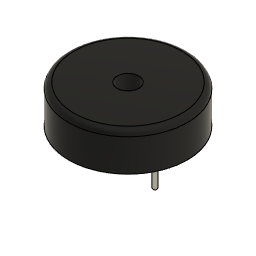
ManvirExam v2 (Autodesk Fusion 360 archive; units mm, degrees)
design "PKM22EPPH4001-B0"
Autodesk Fusion 360 part; units mm, degrees
ref_plane "WorkPlane1" through (0, 0, 1.2) normal (0, 0, 1) x (1, 0, 0) in component "Body"
sketch "Sketch1" plane through (0, 0, 1.2) normal (0, 0, 1) x (1, 0, 0) in component "Body"
  circle A0 centre (0, 0) radius 11
  dimension "d2" = 22
  constraint coincident A0.centre origin
  measures "d2" diameter of A0
extrude "Extrude1" add sketch "Sketch1" along normal blind 7 makes body 1 in component "Body"
fillet "Fillet1" radius 1 1 edges at (-10.2556, -3.9778, 8.2) on bodies 1 in component "Body"
sketch "Sketch2" plane through (0, 0, 1.2) normal (0, 0, -1) x (1, 0, 0) in component "Body"
  circle A0 centre (0, 0) radius 11
  line L0 (0, 11) -> (0, -11) construction
  circle A1 centre (0, 5) radius 0.6
  circle A2 centre (0, -5) radius 0.6
  line L1 (-11, 0) -> (11, 0) construction
  circle A3 centre (-5, 0) radius 1.75
  circle A4 centre (5, 0) radius 1.75
  dimension "d7" = 1.2
  dimension "d8" = 10
  dimension "d9" = 3.5
  dimension "d10" = 10
  constraint coincident A0 L0.start
  constraint coincident A0 L0.end
  constraint vertical L0
  constraint coincident A0.centre L0
  constraint coincident L0 A1.centre
  constraint coincident L0 A2.centre
  constraint equal A1 A2
  constraint coincident A0 L1.start
  constraint coincident A0 L1.end
  constraint coincident A0.centre L1
  constraint horizontal L1
  constraint symmetric A1.centre A2.centre L1
  constraint coincident L1 A3.centre
  constraint coincident L1 A4.centre
  constraint equal A3 A4
  constraint symmetric L0 A3.centre A4.centre
  measures "d7" diameter of A1
  measures "d8" distance of A1.centre A2.centre
  measures "d9" diameter of A3
  measures "d10" distance of A3.centre A4.centre
extrude "Extrude2" add sketch "Sketch2" along normal blind 1.2 contours A1 | A2 | A3 | A4 bodies 1 in component "Body"
chamfer "Chamfer1" distance 0.3 angle 45 2 edges at (-6.6316, 0.6328, 0) (3.3684, 0.6328, 0) on bodies 1 in component "Body"
sketch "Sketch3" plane through (0, 0, 8.2) normal (0, 0, 1) x (-1, 0, 0) in component "Body"
  circle A0 centre (0, 0) radius 10
  circle A1 centre (0, 0) radius 2
  dimension "d14" = 4
  constraint concentric A0 A1
  measures "d14" diameter of A1
extrude "Extrude3" cut sketch "Sketch3" against normal blind 3 contours A1 bodies 1 in component "Body"
extrude "Extrude1'" add 1 faces at (-0.637, -0.1965, 5.2) along direction (0, 0, 1) blind 0.25 separate body on bodies 1 makes body 2 in component "Transducer"
sketch "Sketch1 (2)" plane through (0, 0, 0) normal (0, 0, -1) x (1, 0, 0) in component "Pins"
  circle A0 centre (-5, 0) radius 1.45
  circle A1 centre (-5, 0) radius 1.75
  line L0 (-4.5934, -0.1591) -> (-4.8409, -0.4066)
  line L1 (-4.8409, -0.4066) -> (-5.4066, 0.1591)
  line L2 (-5.4066, 0.1591) -> (-5.1591, 0.4066)
  line L3 (-5.1591, 0.4066) -> (-4.5934, -0.1591)
  line L4 (-4.5934, -0.1591) -> (-5.4066, 0.1591) construction
  line L5 (-4.8409, -0.4066) -> (-5.1591, 0.4066) construction
  line L6 (-5, 0) -> (-5.0493, 0.0193)
  line L7 (-5, 0) -> (-6.75, 0) construction
  line L8 (-5, 0) -> (-6.2374, 1.2374) construction
  circle A2 centre (5, 0) radius 1.75
  line L9 (5, 0) -> (3.25, 0) construction
  line L10 (5, 0) -> (3.7626, 1.2374) construction
  line L11 (5.4066, -0.1591) -> (5.1591, -0.4066)
  line L12 (5.1591, -0.4066) -> (4.5934, 0.1591)
  line L13 (4.5934, 0.1591) -> (4.8409, 0.4066)
  line L14 (4.8409, 0.4066) -> (5.4066, -0.1591)
  line L15 (5.4066, -0.1591) -> (4.5934, 0.1591) construction
  line L16 (5.1591, -0.4066) -> (4.8409, 0.4066) construction
  point P0 (-5, 0)
  point P1 (5, 0)
  dimension "d19" = 0.35
  dimension "d20" = 0.8
  dimension "d21" = 45
  dimension "d24" = 45
  constraint perpendicular L0 L1
  constraint parallel L0 L2
  constraint parallel L1 L3
  constraint coincident L4 P0
  constraint coincident L5 P0
  constraint coincident P0 A0.centre
  constraint coincident L4 L6.end
  constraint parallel L4 L6
  constraint coincident A1 L7.end
  constraint horizontal L7
  constraint coincident A1 L8.end
  constraint symmetric L1.end L2.end L8
  constraint coincident P1 A2.centre
  constraint coincident A2 L9.end
  constraint horizontal L9
  constraint coincident A2 L10.end
  constraint perpendicular L11 L12
  constraint parallel L11 L13
  constraint parallel L12 L14
  constraint coincident L15 P1
  constraint coincident L16 P1
  constraint equal L1 L12
  constraint equal L2 L13
  constraint symmetric L10 L12.end L13.end
  measures "d19" distance of L1.end L2.end
  measures "d20" distance of L0.end L1.end
  measures "d21" angle of L7 L8
  measures "d24" angle of L9 L10
extrude "Extrude1''" add sketch "Sketch1 (2)" along normal blind 6.5 separate body contours L0 L1 L2 L3 | L11 L12 L13 L14 makes body 3 at (-5.0295, 0.218, -2.1667) makes body 4 at (4.9705, 0.218, -2.1667) in component "Pins"
chamfer "Chamfer1'" distance 0.3 angle 45 4 edges at (4.7172, -0.2828, -6.5) (5.2828, 0.2828, -6.5) (-5.2828, -0.2828, -6.5) (-4.7172, 0.2828, -6.5) on bodies 3 4 in component "Pins"
component "Body" placed x (1, 0, 0) y (0, 1, 0) z (0, 0, 1) at (0, 0, 0)
component "Transducer" placed x (1, 0, 0) y (0, 1, 0) z (0, 0, 1) at (0, 0, 0)
component "Pins" placed x (1, 0, 0) y (0, 1, 0) z (0, 0, 1) at (0, 0, 0)
equation "d24 = d21"
